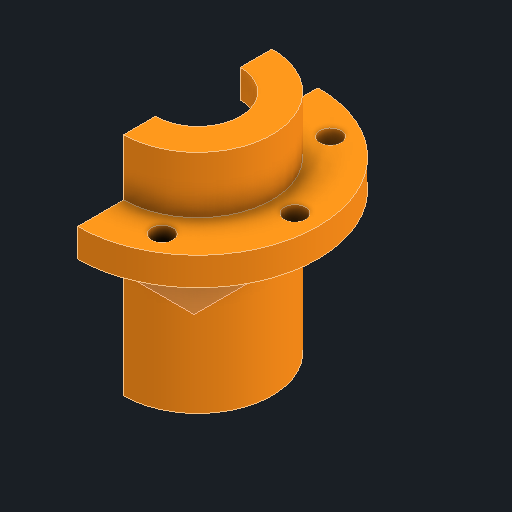
# Autodesk Inventor part: Bearing_Holder
Saved by Autodesk Inventor 2024.1 (Build 281209000, 209)
## iProperties
Created: 2023-08-03
Part Number: Bearing_Holder
Material: PC/ABS Plastic
Document SubType Name: Modeling
Designer: jaege
Density: 1.1 g/cm^3
Appearance: Orange
Author: jaege
Autodesk Inventor part; units mm, degrees
ref_plane "YZ Plane" through (0, 0, 0) normal (1, 0, 0) x (0, 1, 0)
ref_plane "XZ Plane" through (0, 0, 0) normal (0, 1, 0) x (-1, 0, 0)
ref_plane "XY Plane" through (0, 0, 0) normal (0, 0, 1) x (1, 0, 0)
sketch "Sketch1" plane through (0, 0, 0) normal (0, 1, 0) x (-1, 0, 0)
  arc A0 (0, 7.5) -> (0, -7.5) centre (0, 0) ccw
  arc A1 (0, 10.5) -> (0, -10.5) centre (0, 0) ccw
  line L0 (0, 10.5) -> (0, 7.5)
  line L1 (0, -7.5) -> (0, -10.5)
  dimension "d0" = 7.5
  dimension "d1" = 3
  constraints: 4 end point, 4 point on circle, 2 centre point, 2 vertical, 2 vertical alignment, 1 coincident
  measures "d0" radius of A0
  measures "d1" radial gap between concentric circles of A0 A1
extrude "Extrusion1" add sketch "Sketch1" along normal blind 24
sketch "Sketch2" plane through (0, 24, 0) normal (0, 1, 0) x (1, 0, 0)
  line L0 (0, 10.5) -> (0, 7.5) projected
  line L1 (0, -7.5) -> (0, -10.5) projected
  arc A0 (0, -10.5) -> (0, 10.5) centre (0, 0) ccw projected
  arc A1 (0, -6) -> (0, 6) centre (0, 0) ccw
  line L2 (0, 0) -> (0, 6) construction
  line L3 (0, 0) -> (6, 0) construction
  line L4 (0, 0) -> (0, -6) construction
  line L5 (0, 6) -> (0, 10.5)
  line L6 (0, -6) -> (0, -10.5)
  dimension "d6" = 6
  dimension "d7" = 90
  dimension "d8" = 180
  constraints: 10 end point, 2 point on circle, 1 centre point, 1 coincident, 1 horizontal, 1 perpendicular
  measures "d6" radius of A1
  measures "d7" angle of L3 L2
  measures "d8" angle of L4 L2
extrude "Extrusion2" add sketch "Sketch2" along normal blind 4
sketch "Sketch3" plane through (0, 0, 0) normal (0, -1, 0) x (1, 0, 0)
  line L0 (0, -10.5) -> (0, -6) projected
  arc A0 (0, -6) -> (0, 6) centre (0, 0) ccw projected
  line L1 (0, 6) -> (0, 10.5) projected
  arc A1 (0, -10.5) -> (0, 10.5) centre (0, 0) ccw projected
extrude "Extrusion3" add sketch "Sketch3" along normal blind 4
ref_plane "Work Plane2" through (0, 16, 0) normal (0, 1, 0) x (1, 0, 0)
ref_plane "Work Plane1" through (0, 12, 0) normal (0, 1, 0) x (1, 0, 0)
sketch "Sketch5" plane through (0, 16, 0) normal (0, 1, 0) x (1, 0, 0)
  arc A0 (0, -10.5) -> (0, 10.5) centre (0, 0) ccw projected
  arc A1 (0, -17) -> (0, 17) centre (0, 0) ccw
  line L0 (0, 10.5) -> (0, 6) projected
  line L1 (0, 17) -> (0, 10.5)
  line L2 (0, -10.5) -> (0, -17)
  circle A2 centre (13.75, 0) radius 1.5
  line L3 (10.5, 0) -> (17, 0) construction
  circle A3 centre (6.875, 11.9078) radius 1.5
  circle A4 centre (6.875, -11.9078) radius 1.5
  dimension "d22" = 6.5
  dimension "d23" = 3
  dimension "d26" = 60
  dimension "d30" = 60
  constraints: 6 end point, 4 centre point, 4 point on circle, 1 collinear, 1 midpoint, 1 vertical, 6 other
  measures "d22" radial gap between concentric circles of A0 A1
  measures "d23" diameter of A2
extrude "Extrusion4" add sketch "Sketch5" along normal blind 4
body "Solid1"
